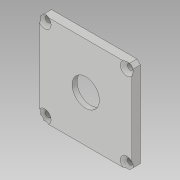
# Autodesk Inventor part: bearing_mount_part_2
Saved by Autodesk Inventor 2017 (Build 210142000, 142)
## iProperties
Part Number: bearing_mount_part_2
Material: Generisch
Document SubType Name: Modeling
Designer: Max
Density: 1 g/cm^3
Appearance: Vorgabe
Author: Max
Autodesk Inventor part; units mm, degrees
ref_plane "YZ Plane" through (0, 0, 0) normal (1, 0, 0) x (0, 1, 0)
ref_plane "XZ Plane" through (0, 0, 0) normal (0, 1, 0) x (-1, 0, 0)
ref_plane "XY Plane" through (0, 0, 0) normal (0, 0, 1) x (1, 0, 0)
sketch "Skizze1" plane through (0, 0, 0) normal (0, 1, 0) x (-1, 0, 0)
  line L0 (-27, 27) -> (27, 27)
  line L1 (27, 27) -> (27, -27)
  line L2 (27, -27) -> (-27, -27)
  line L3 (-27, -27) -> (-27, 27)
  line L4 (-27, 27) -> (27, -27) construction
  line L5 (27, 27) -> (-27, -27) construction
  point P0 (0, 0)
  dimension "d0" = 54
  dimension "d1" = 54
  constraints: 12 end point, 2 midpoint, 2 parallel, 1 horizontal, 1 perpendicular
  measures "d0" distance of L1.end L2.end
  measures "d1" distance of L0.end L1.end
extrude "Extrusion1" add sketch "Skizze1" along normal blind 5
chamfer "Fase1" distance 2 angle 45 4 edges at (27, 2.5, 27) (27, 2.5, -27) (-27, 2.5, 27) (-27, 2.5, -27)
sketch "Skizze2" plane through (0, 5, 0) normal (0, 1, 0) x (1, 0, 0)
  circle A0 centre (0, 0) radius 11
  dimension "d7" = 22
  constraints: 1 centre point, 1 coincident
  measures "d7" diameter of A0
extrude "Extrusion2" cut sketch "Skizze2" against normal blind 2.1
sketch "Skizze5" plane through (0, 0, 0) normal (0, -1, 0) x (1, 0, 0)
  line L0 (-24, -24) -> (24, -24)
  line L1 (24, -24) -> (24, 24)
  line L2 (24, 24) -> (-24, 24)
  line L3 (-24, 24) -> (-24, -24)
  line L4 (-24, -24) -> (24, 24) construction
  line L5 (24, -24) -> (-24, 24) construction
  point P0 (0, 0)
  dimension "d22" = 48
  dimension "d23" = 48
  constraints: 12 end point, 2 midpoint, 2 parallel, 1 horizontal, 1 perpendicular
  measures "d22" distance of L1.end L2.end
  measures "d23" distance of L0.end L1.end
hole "Bohrung2" at (-24, 0, -24) at (-24, 0, 24) at (24, 0, 24) at (24, 0, -24) direction (0, 1, 0) diameter 3.4 depth 10.688 tip angle 118 countersink diameter 7.5 countersink angle 90 clearance for "Innensechskant-Senkkopfschraube ISO 10642" size "M3" standard "ISO"
sketch "Skizze6" plane through (0, 0, 0) normal (0, -1, 0) x (1, 0, 0)
  circle A0 centre (0, 0) radius 8
  dimension "d31" = 16
  constraints: 1 centre point, 1 coincident
  measures "d31" diameter of A0
extrude "Extrusion4" cut sketch "Skizze6" against normal through all
